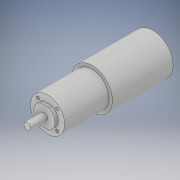
# Autodesk Inventor part: 12RPM Gear Motor
Saved by Autodesk Inventor 2017 (Build 210142000, 142)
## iProperties
Created: 2018-10-09
Part Number: 12RPM Gear Motor
Material: Generic
Document SubType Name: Modeling
Designer: Zach
Density: 1 g/cm^3
Appearance: Default
Author: Zach
Autodesk Inventor part; units mm, degrees
ref_plane "YZ Plane" through (0, 0, 0) normal (1, 0, 0) x (0, 1, 0)
ref_plane "XZ Plane" through (0, 0, 0) normal (0, 1, 0) x (-1, 0, 0)
ref_plane "XY Plane" through (0, 0, 0) normal (0, 0, 1) x (1, 0, 0)
sketch "Sketch1" plane through (0, 0, 0) normal (0, 0, 1) x (1, 0, 0)
  circle A0 centre (0, 0) radius 19
  dimension "d0" = 38
  constraints: 1 centre point, 1 coincident
  measures "d0" diameter of A0
extrude "Extrusion1" add sketch "Sketch1" along normal blind 57.1
sketch "Sketch2" plane through (0, 0, 57.1) normal (0, 0, 1) x (1, 0, 0)
  circle A0 centre (0, 0) radius 16
  dimension "d3" = 32
  constraints: 1 centre point, 1 coincident
  measures "d3" diameter of A0
extrude "Extrusion2" add sketch "Sketch2" along normal blind 41.8
sketch "Sketch3" plane through (0, 0, 98.9) normal (0, 0, 1) x (1, 0, 0)
  circle A0 centre (0, 0) radius 10
  dimension "d6" = 20
  constraints: 1 centre point, 1 coincident
  measures "d6" diameter of A0
extrude "Extrusion3" add sketch "Sketch3" along normal blind 3
sketch "Sketch4" plane through (0, 0, 101.9) normal (0, 0, 1) x (1, 0, 0)
  circle A0 centre (0, 0) radius 3
  dimension "d9" = 6
  constraints: 1 centre point, 1 coincident
  measures "d9" diameter of A0
extrude "Extrusion4" add sketch "Sketch4" along normal blind 16.2
sketch "Sketch5" plane through (0, 0, 101.9) normal (0, 0, 1) x (1, 0, 0)
  line L0 (-9, -9) -> (9, -9) construction
  line L1 (9, -9) -> (9, 9) construction
  line L2 (9, 9) -> (-9, 9) construction
  line L3 (-9, 9) -> (-9, -9) construction
  line L4 (-9, -9) -> (9, 9) construction
  line L5 (9, -9) -> (-9, 9) construction
  circle A0 centre (9, 9) radius 1.5
  circle A1 centre (9, -9) radius 1.5
  circle A2 centre (-9, -9) radius 1.5
  circle A3 centre (-9, 9) radius 1.5
  point P0 (0, 0)
  dimension "d12" = 18
  dimension "d13" = 18
  dimension "d14" = 3
  dimension "d15" = 3
  dimension "d16" = 3
  dimension "d17" = 3
  constraints: 12 end point, 4 centre point, 4 coincident, 2 midpoint, 2 parallel, 1 horizontal, 1 perpendicular
  measures "d12" distance of L2.end L1.end
  measures "d13" distance of L1.end L0.end
  measures "d14" diameter of A0
  measures "d15" diameter of A1
  measures "d16" diameter of A2
  measures "d17" diameter of A3
extrude "Extrusion5" cut sketch "Sketch5" against normal blind 25
sketch "Sketch6" plane through (0, 0, 98.9) normal (0, 0, 1) x (1, 0, 0)
  circle A0 centre (0, 0) radius 3 projected
  circle A1 centre (0, 0) radius 10 projected
  line L0 (-4.3589, -9) -> (4.3589, -9)
  line L1 (-4.3589, 9) -> (4.3589, 9)
  dimension "d20" = 18
  constraints: 4 end point, 4 point on circle, 1 horizontal, 1 parallel, 1 vertical alignment
  measures "d20" distance between parallel lines of L0 L1
extrude "Extrusion6" cut sketch "Sketch6" along normal through all contours L1 A1 | A1 L0
body "Solid1"
